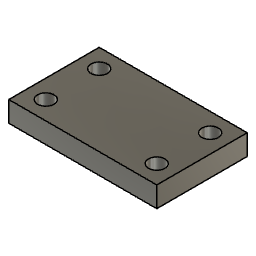
Chip -- Editable (Autodesk Fusion 360 archive; units mm, degrees)
design "PMMA"
Autodesk Fusion 360 part; units mm, degrees
sketch "Sketch1" plane through (0, 0, 0) normal (0, 0, 1) x (1, 0, 0)
  line L0 (10, 25) -> (46, 25)
  line L1 (46, 25) -> (46, 3)
  line L2 (46, 3) -> (10, 3)
  line L3 (10, 3) -> (10, 25)
  dimension "d1" = 36
  dimension "d2" = 22
  constraint horizontal L0
  constraint vertical L1
  constraint horizontal L2
  constraint vertical L3
  measures "d1" distance of L0.start L0.end
  measures "d2" distance of L0.start L2.end
extrude "Extrude1" add sketch "Sketch1" along normal blind 5
sketch "Sketch2" plane through (0, 0, 5) normal (0, 0, 1) x (-1, 0, 0)
  line L0 (-10, -3) -> (-46, -3)
  line L1 (-46, -3) -> (-46, -25)
  line L2 (-46, -25) -> (-10, -25)
  line L3 (-10, -25) -> (-10, -3)
  line L4 (-21.9549, -14.5099) -> (-33.9998, -14.5099)
  line L5 (-33.9998, -14.5099) -> (-33.9998, -13.5007)
  line L6 (-33.9998, -13.5007) -> (-21.9549, -13.5007)
  line L7 (-21.9549, -13.5007) -> (-21.9549, -14.5099)
  constraint horizontal L4
  constraint vertical L5
  constraint horizontal L6
  constraint vertical L7
hole "Hole3" at (14.5003, 20.5001, 5) direction (0, 0, -1) diameter 4 depth 5 tip angle 180
pattern_linear "R-Pattern2" count 2 spacing 13 along (0, -1, 0) count 2 spacing 27 along (1, 0, 0) of "Hole3"

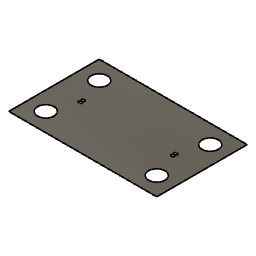
design "Membrane"
Autodesk Fusion 360 part; units mm, degrees
sketch "Sketch1" plane through (0, 0, 0) normal (0, 0, 1) x (1, 0, 0)
  line L0 (10, 25) -> (46, 25)
  line L1 (46, 25) -> (46, 3)
  line L2 (46, 3) -> (10, 3)
  line L3 (10, 3) -> (10, 25)
  dimension "d1" = 36
  dimension "d2" = 22
  constraint horizontal L0
  constraint vertical L1
  constraint horizontal L2
  constraint vertical L3
  measures "d1" distance of L0.start L0.end
  measures "d2" distance of L0.start L2.end
extrude "Extrude1" add sketch "Sketch1" along normal blind 0.05
sketch "Sketch5" plane through (0, 0, 0.05) normal (0, 0, 1) x (-1, 0, 0)
  line L0 (-10, -3) -> (-46, -3)
  line L1 (-46, -3) -> (-46, -25)
  line L2 (-46, -25) -> (-10, -25)
  line L3 (-10, -25) -> (-10, -3)
  line L4 (-16.7182, -15.0406) -> (-21.9549, -13.5007)
  line L5 (-21.9549, -14.5099) -> (-16.0325, -16.2515)
  line L6 (-16.7182, -15.0406) -> (-16.0325, -16.2515)
  constraint parallel L4 L5
hole "Hole3" at (14.5003, 20.5001, 0.05) direction (0, 0, -1) diameter 4 depth 4 tip angle 180
pattern_linear "R-Pattern2" count 2 spacing 13 along (0, -1, 0) count 2 spacing 27 along (1, 0, 0) of "Hole3"
sketch "Sketch11" plane through (0, 0, 0.05) normal (0, 0, 1) x (-1, 0, 0)
  circle A0 centre (-41.5003, -7.5001) radius 2
  circle A1 centre (-41.5003, -20.5001) radius 2
  circle A2 centre (-14.5003, -7.5001) radius 2
  circle A3 centre (-14.5003, -20.5001) radius 2
  line L0 (-10, -3) -> (-46, -3)
  line L1 (-46, -3) -> (-46, -25)
  line L2 (-46, -25) -> (-10, -25)
  line L3 (-10, -25) -> (-10, -3)
  line L4 (-16.3501, -14.6002) -> (-17.1489, -14.6002)
  line L5 (-17.1489, -14.6002) -> (-17.1489, -14.1)
  line L6 (-17.1489, -14.1) -> (-16.3501, -14.1)
  line L7 (-16.3501, -14.1) -> (-16.3501, -14.6002)
  line L8 (-16.3495, -13.4) -> (-17.1505, -13.4)
  line L9 (-17.1505, -13.4) -> (-17.1505, -13.9)
  line L10 (-17.1505, -13.9) -> (-16.3495, -13.9)
  line L11 (-16.3495, -13.9) -> (-16.3495, -13.4)
  constraint horizontal L4
  constraint vertical L5
  constraint horizontal L6
  constraint vertical L7
  constraint horizontal L8
  constraint vertical L9
  constraint horizontal L10
  constraint vertical L11
extrude "Extrude8" cut sketch "Sketch11" against normal blind 1.6 contours L4 L5 L6 L7 | L8 L9 L10 L11
sketch "Sketch15" plane through (0, 0, 0.05) normal (0, 0, 1) x (-1, 0, 0)
  line L0 (-16.3495, -13.4) -> (-16.3495, -13.9)
  line L1 (-16.3495, -13.9) -> (-17.1505, -13.9)
  line L2 (-17.1505, -13.9) -> (-17.1505, -13.4)
  line L3 (-17.1505, -13.4) -> (-16.3495, -13.4)
  line L4 (-16.3501, -14.6002) -> (-17.1489, -14.6002)
  line L5 (-17.1489, -14.6002) -> (-17.1489, -14.1)
  line L6 (-17.1489, -14.1) -> (-16.3501, -14.1)
  line L7 (-16.3501, -14.1) -> (-16.3501, -14.6002)
  circle A0 centre (-41.5003, -7.5001) radius 2
  circle A1 centre (-41.5003, -20.5001) radius 2
  circle A2 centre (-14.5003, -7.5001) radius 2
  circle A3 centre (-14.5003, -20.5001) radius 2
  line L8 (-10, -3) -> (-46, -3)
  line L9 (-46, -3) -> (-46, -25)
  line L10 (-46, -25) -> (-10, -25)
  line L11 (-10, -25) -> (-10, -3)
  line L12 (-38.8493, -14.6007) -> (-39.6492, -14.6007)
  line L13 (-39.6492, -14.6007) -> (-39.6492, -14.1)
  line L14 (-39.6492, -14.1) -> (-38.8493, -14.1)
  line L15 (-38.8493, -14.1) -> (-38.8493, -14.6007)
  line L16 (-38.8501, -13.9) -> (-39.65, -13.9)
  line L17 (-39.65, -13.9) -> (-39.65, -13.3997)
  line L18 (-39.65, -13.3997) -> (-38.8501, -13.3997)
  line L19 (-38.8501, -13.3997) -> (-38.8501, -13.9)
  constraint horizontal L12
  constraint vertical L13
  constraint horizontal L14
  constraint vertical L15
  constraint horizontal L16
  constraint vertical L17
  constraint horizontal L18
  constraint vertical L19
extrude "Extrude10" cut sketch "Sketch15" against normal blind 1.6 contours L12 L13 L14 L15 | L16 L17 L18 L19
